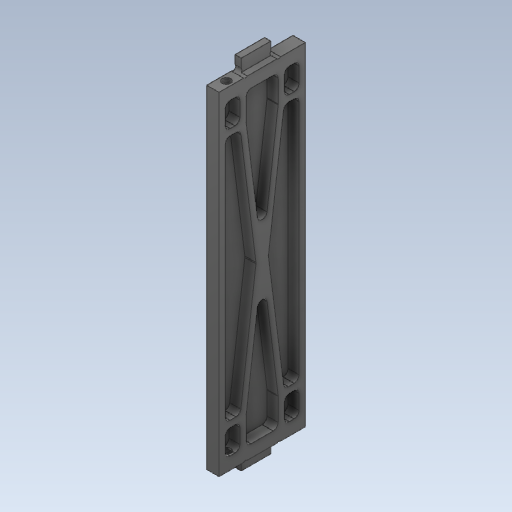
# Autodesk Inventor part: Cockpit_battery_front_frame
Saved by Autodesk Inventor 2020.4 (Build 244396000, 396)
## iProperties
Created: 2022-01-28
Part Number: Cockpit_battery_front_frame
Material: アセタール樹脂、黒
Document SubType Name: Modeling
Designer: Masato Kubotera
Density: 1.425 g/cm^3
Appearance: 滑らか - 黒
Description: POM T5
Author: Masato Kubotera
Autodesk Inventor part; units mm, degrees
ref_plane "XZ Plane" through (0, 0, 0) normal (0, 1, 0) x (-1, 0, 0)
ref_plane "XY Plane" through (0, 0, 0) normal (0, 0, 1) x (1, 0, 0)
derived "Cockpit_side_frame.ipt"
sketch "スケッチ2" plane through (0, 0, 0) normal (0, 1, 0) x (-1, 0, 0)
  line L0 (-28.5, -22.5) -> (88.5, -22.5) construction
  line L1 (88.5, -22.5) -> (88.5, -138.5)
  line L2 (88.5, -96) -> (-28.5, -96) construction
  line L3 (-28.5, -96) -> (-28.5, -22.5) construction
  line L4 (-28.5, -22.5) -> (88.5, -96) construction
  line L5 (88.5, -22.5) -> (-28.5, -96) construction
  line L6 (38.5, -101) -> (38.5, -133.5)
  line L7 (43.5, -138.5) -> (88.5, -138.5)
  arc A0 (64.6349, -63.15) -> (63.15, -64.6349) centre (63.8925, -63.8925) ccw
  arc A1 (73.15, -65.2849) -> (71.6651, -63.8) centre (72.4075, -64.5425) ccw
  line L8 (65.3349, -63.8) -> (71.6651, -63.8)
  line L9 (64.6349, -63.15) -> (72.3651, -63.15)
  line L10 (63.9, -63.85) -> (73.1, -63.85) construction
  arc A2 (65.3349, -63.8) -> (63.85, -65.2849) centre (64.5925, -64.5425) ccw
  line L11 (63.2, -63.2) -> (73.8, -63.2) construction
  line L12 (73.15, -65.2849) -> (73.15, -76.2151)
  line L13 (73.8, -70.75) -> (63.2, -70.75) construction
  line L14 (73.85, -64.6349) -> (73.85, -76.8651)
  line L15 (73.1, -63.85) -> (73.1, -77.65) construction
  line L16 (63.85, -65.2849) -> (63.85, -76.2151)
  line L17 (73.8, -63.2) -> (73.8, -78.3) construction
  line L18 (63.15, -64.6349) -> (63.15, -76.8651)
  line L19 (68.5, -63.2) -> (68.5, -78.3) construction
  line L20 (63.9, -77.65) -> (63.9, -63.85) construction
  line L21 (73.1, -63.85) -> (63.9, -77.65) construction
  line L22 (73.8, -63.2) -> (63.2, -78.3) construction
  line L23 (63.2, -63.2) -> (73.8, -78.3) construction
  line L24 (63.2, -78.3) -> (63.2, -63.2) construction
  line L25 (63.9, -63.85) -> (73.1, -77.65) construction
  arc A3 (73.85, -64.6349) -> (72.3651, -63.15) centre (73.1075, -63.8925) ccw
  line L26 (73.1, -77.65) -> (63.9, -77.65) construction
  line L27 (73.8, -78.3) -> (63.2, -78.3) construction
  arc A4 (63.85, -76.2151) -> (65.3349, -77.7) centre (64.5925, -76.9575) ccw
  arc A5 (63.15, -76.8651) -> (64.6349, -78.35) centre (63.8925, -77.6075) ccw
  line L28 (65.3349, -77.7) -> (71.6651, -77.7)
  line L29 (64.6349, -78.35) -> (72.3651, -78.35)
  arc A6 (71.6651, -77.7) -> (73.15, -76.2151) centre (72.4075, -76.9575) ccw
  arc A7 (72.3651, -78.35) -> (73.85, -76.8651) centre (73.1075, -77.6075) ccw
  line L30 (-23.5, -22.5) -> (-28.5, -27.5)
  line L31 (-28.5, -59.25) -> (88.5, -59.25) construction
  line L32 (30, -22.5) -> (30, -96) construction
  line L33 (-23.5, -96) -> (-28.5, -91)
  line L34 (-28.5, -27.5) -> (-28.5, -91)
  line L35 (-20.5, -24.5) -> (-25.5, -24.5) construction
  line L36 (-25.5, -24.5) -> (-25.5, -94) construction
  line L37 (-25.5, -94) -> (-20.5, -94) construction
  line L38 (-20.5, -94) -> (-20.5, -24.5) construction
  line L39 (-20.5, -24.5) -> (-25.5, -94) construction
  line L40 (-25.5, -24.5) -> (-20.5, -94) construction
  line L41 (-25.55, -46.7) -> (-20.45, -46.7)
  line L42 (-20.45, -46.7) -> (-20.45, -71.8)
  line L43 (-20.45, -71.8) -> (-25.55, -71.8)
  line L44 (-25.55, -71.8) -> (-25.55, -46.7)
  line L45 (-25.55, -46.7) -> (-20.45, -71.8) construction
  line L46 (-20.45, -46.7) -> (-25.55, -71.8) construction
  line L47 (-25.5, -46.75) -> (-20.5, -46.75) construction
  line L48 (-25.5, -71.75) -> (-20.5, -71.75) construction
  line L49 (-23, -24.5) -> (-23, -94) construction
  circle A8 centre (-23, -35) radius 3
  circle A9 centre (-23, -35) radius 1.6
  arc A10 (-24.0651, -46.7) -> (-25.55, -48.1849) centre (-24.8075, -47.4425) ccw
  arc A11 (-20.45, -48.1849) -> (-21.9349, -46.7) centre (-21.1925, -47.4425) ccw
  arc A12 (-21.9349, -71.8) -> (-20.45, -70.3151) centre (-21.1925, -71.0575) ccw
  arc A13 (-25.55, -70.3151) -> (-24.0651, -71.8) centre (-24.8075, -71.0575) ccw
  circle A14 centre (-23, -83.5) radius 1.6
  circle A15 centre (-23, -83.5) radius 3
  line L50 (33.5, -96) -> (38.5, -101)
  line L51 (-23.5, -96) -> (33.5, -96)
  line L52 (81, -46.5) -> (-20.5, -46.5) construction
  line L53 (-20.5, -46.5) -> (-20.5, -41.5) construction
  line L54 (-20.5, -41.5) -> (81, -41.5) construction
  line L55 (81, -41.5) -> (81, -46.5) construction
  line L56 (81, -46.5) -> (-20.5, -41.5) construction
  line L57 (-20.5, -46.5) -> (81, -41.5) construction
  line L58 (-20.5, -44) -> (81, -44) construction
  line L59 (30.25, -41.5) -> (30.25, -46.5) construction
  line L60 (5.25, -41.5) -> (5.25, -46.5) construction
  line L61 (55.3, -41.45) -> (5.2, -41.45)
  line L62 (5.2, -41.45) -> (5.2, -46.55)
  line L63 (5.2, -46.55) -> (55.3, -46.55)
  line L64 (55.3, -46.55) -> (55.3, -41.45)
  line L65 (55.3, -41.45) -> (5.2, -46.55) construction
  line L66 (5.2, -41.45) -> (55.3, -46.55) construction
  arc A16 (6.6849, -41.45) -> (5.2, -42.9349) centre (5.9425, -42.1925) ccw
  circle A17 centre (-2.25, -44) radius 3
  circle A18 centre (-2.25, -44) radius 1.6
  line L67 (55.25, -41.5) -> (55.25, -46.5) construction
  arc A19 (55.3, -42.9349) -> (53.8151, -41.45) centre (54.5575, -42.1925) ccw
  circle A20 centre (62.75, -44) radius 3
  circle A21 centre (62.75, -44) radius 1.6
  arc A22 (5.2, -45.0651) -> (6.6849, -46.55) centre (5.9425, -45.8075) ccw
  arc A23 (53.8151, -46.55) -> (55.3, -45.0651) centre (54.5575, -45.8075) ccw
  line L68 (-20.5, -89) -> (81, -89) construction
  line L69 (81, -89) -> (81, -94) construction
  line L70 (81, -94) -> (-20.5, -94) construction
  line L71 (-20.5, -94) -> (-20.5, -89) construction
  line L72 (-20.5, -89) -> (81, -94) construction
  line L73 (81, -89) -> (-20.5, -94) construction
  line L74 (-20.5, -91.5) -> (81, -91.5) construction
  line L75 (30.25, -89) -> (30.25, -94) construction
  line L76 (55.3, -91.55) -> (5.2, -91.55)
  line L77 (5.2, -91.55) -> (5.2, -88.95)
  line L78 (5.2, -88.95) -> (55.3, -88.95)
  line L79 (55.3, -88.95) -> (55.3, -91.55)
  line L80 (55.3, -91.55) -> (5.2, -88.95) construction
  line L81 (5.2, -91.55) -> (55.3, -88.95) construction
  line L82 (5.25, -89) -> (5.25, -91.5) construction
  line L83 (55.25, -89) -> (55.25, -91.5) construction
  line L84 (5.25, -90.25) -> (55.25, -90.25) construction
  arc A24 (7.3, -88.95) -> (5.2, -88.95) centre (6.25, -88.95) ccw
  arc A25 (55.3, -88.95) -> (53.2, -88.95) centre (54.25, -88.95) ccw
  arc A26 (53.2, -91.55) -> (55.3, -91.55) centre (54.25, -91.55) ccw
  arc A27 (5.2, -91.55) -> (7.3, -91.55) centre (6.25, -91.55) ccw
  circle A28 centre (-2.5, -91.5) radius 3
  circle A29 centre (-2.5, -91.5) radius 1.6
  circle A30 centre (62.5, -91.5) radius 3 construction
  circle A31 centre (62.5, -91.5) radius 1.6 construction
  line L85 (-23.5, -22.5) -> (63.7651, -22.5)
  line L86 (65.25, -21.0151) -> (65.25, -17.5)
  line L87 (65.25, -17.5) -> (73.25, -17.5)
  line L88 (73.25, -17.5) -> (73.25, -21.0151)
  line L89 (81, -22.5) -> (81, -17.5)
  line L90 (88.5, -22.5) -> (88.5, -20)
  line L91 (81, -17.5) -> (86, -17.5)
  line L92 (86, -17.5) -> (88.5, -20)
  line L93 (69.25, -17.5) -> (69.25, -22.5) construction
  arc A32 (63.7651, -22.5) -> (65.25, -21.0151) centre (64.5075, -21.7575) ccw
  arc A33 (73.25, -21.0151) -> (74.7349, -22.5) centre (73.9925, -21.7575) ccw
  arc A34 (79.5151, -22.5) -> (81, -21.0151) centre (80.2575, -21.7575) ccw
  line L94 (-15.5, -89) -> (-15.5, -69) construction
  line L95 (-15.5, -69) -> (64.5, -69) construction
  line L96 (64.5, -69) -> (64.5, -89) construction
  line L97 (45.5, -84) -> (-16.5, -84)
  line L98 (-18.5, -82) -> (-18.5, -63.3955)
  line L99 (-16.5, -61.3955) -> (45.5, -61.3955)
  line L100 (47.5, -63.3955) -> (47.5, -82)
  line L101 (47.5, -84) -> (-18.5, -61.3955) construction
  line L102 (-18.5, -84) -> (47.5, -61.3955) construction
  arc A35 (-16.5, -61.3955) -> (-18.5, -63.3955) centre (-16.5, -63.3955) ccw
  arc A36 (-18.5, -82) -> (-16.5, -84) centre (-16.5, -82) ccw
  arc A37 (45.5, -84) -> (47.5, -82) centre (45.5, -82) ccw
  arc A38 (47.5, -63.3955) -> (45.5, -61.3955) centre (45.5, -63.3955) ccw
  line L103 (38.5, -133.5) -> (43.5, -138.5)
  line L104 (46, -131) -> (41, -131) construction
  line L105 (41, -131) -> (41, -96) construction
  line L106 (41, -96) -> (46, -96) construction
  line L107 (46, -96) -> (46, -131) construction
  line L108 (46, -131) -> (41, -96) construction
  line L109 (41, -131) -> (46, -96) construction
  line L110 (43.5, -96) -> (43.5, -131) construction
  line L111 (41, -113.5) -> (46, -113.5) construction
  line L112 (43.5, -107.5) -> (46, -107.5) construction
  line L113 (43.45, -107.45) -> (46.05, -107.45)
  line L114 (46.05, -107.45) -> (46.05, -119.55)
  line L115 (46.05, -119.55) -> (43.45, -119.55)
  line L116 (43.45, -119.55) -> (43.45, -107.45)
  line L117 (43.45, -107.45) -> (46.05, -119.55) construction
  line L118 (46.05, -107.45) -> (43.45, -119.55) construction
  arc A39 (46.05, -109.55) -> (46.05, -107.45) centre (46.05, -108.5) ccw
  arc A40 (44.9349, -107.45) -> (43.45, -108.9349) centre (44.1925, -108.1925) ccw
  arc A41 (46.05, -119.55) -> (46.05, -117.45) centre (46.05, -118.5) ccw
  line L119 (43.5, -119.5) -> (46, -119.5) construction
  arc A42 (43.45, -118.0651) -> (44.9349, -119.55) centre (44.1925, -118.8075) ccw
  line L120 (44.75, -107.5) -> (44.75, -119.5) construction
  circle A43 centre (43.5, -125.5) radius 3 construction
  circle A44 centre (43.5, -125.5) radius 1.6 construction
  circle A45 centre (43.5, -101.5) radius 3
  circle A46 centre (43.5, -101.5) radius 1.6
  circle A47 centre (-13.5, -55) radius 2
  line L121 (41, -131) -> (79.8645, -131) construction
  line L122 (79.8645, -131) -> (79.8645, -136) construction
  line L123 (79.8645, -136) -> (41, -136) construction
  line L124 (41, -136) -> (41, -131) construction
  line L125 (41, -131) -> (79.8645, -136) construction
  line L126 (79.8645, -131) -> (41, -136) construction
  line L127 (41, -133.5) -> (79.8645, -133.5) construction
  line L128 (60.4322, -131) -> (60.4322, -136) construction
  line L129 (60.4322, -133.5) -> (60.4322, -131) construction
  line L130 (52.8822, -130.95) -> (67.9822, -130.95)
  line L131 (67.9822, -130.95) -> (67.9822, -133.55)
  line L132 (67.9822, -133.55) -> (52.8822, -133.55)
  line L133 (52.8822, -133.55) -> (52.8822, -130.95)
  line L134 (52.8822, -130.95) -> (67.9822, -133.55) construction
  line L135 (67.9822, -130.95) -> (52.8822, -133.55) construction
  line L136 (52.9322, -131) -> (52.9322, -133.5) construction
  arc A48 (54.9822, -130.95) -> (52.8822, -130.95) centre (53.9322, -130.95) ccw
  arc A49 (52.8822, -132.0651) -> (54.3672, -133.55) centre (53.6247, -132.8075) ccw
  arc A50 (67.9822, -130.95) -> (65.8822, -130.95) centre (66.9322, -130.95) ccw
  arc A51 (66.4973, -133.55) -> (67.9822, -132.0651) centre (67.2398, -132.8075) ccw
  line L137 (67.9322, -131) -> (67.9322, -133.5) construction
  line L138 (52.9322, -132.25) -> (67.9322, -132.25) construction
  circle A52 centre (74.4322, -133.5) radius 1.6 construction
  circle A53 centre (74.4322, -133.5) radius 3 construction
  circle A54 centre (46.4322, -133.5) radius 3
  circle A55 centre (46.4322, -133.5) radius 1.6
  line L139 (50.5, -96.5) -> (79, -96.5)
  line L140 (81, -98.5) -> (81, -126.5)
  line L141 (79, -128.5) -> (50.5, -128.5)
  line L142 (48.5, -126.5) -> (48.5, -98.5)
  line L143 (48.5, -96.5) -> (81, -128.5) construction
  line L144 (81, -96.5) -> (48.5, -128.5) construction
  arc A56 (50.5, -96.5) -> (48.5, -98.5) centre (50.5, -98.5) ccw
  arc A57 (48.5, -126.5) -> (50.5, -128.5) centre (50.5, -126.5) ccw
  arc A58 (79, -128.5) -> (81, -126.5) centre (79, -126.5) ccw
  arc A59 (81, -98.5) -> (79, -96.5) centre (79, -98.5) ccw
  line L145 (81, -91.6746) -> (86, -91.6746) construction
  line L146 (86, -91.6746) -> (86, -136) construction
  line L147 (86, -136) -> (81, -136) construction
  line L148 (81, -136) -> (81, -91.6746) construction
  line L149 (81, -91.6746) -> (86, -136) construction
  line L150 (86, -91.6746) -> (81, -136) construction
  line L151 (83.5, -91.6746) -> (83.5, -136) construction
  circle A60 centre (83.5, -94.1746) radius 1.475
  circle A61 centre (83.5, -99.1746) radius 1.475
  circle A62 centre (83.5, -104.1746) radius 1.475
  circle A63 centre (83.5, -133.5) radius 1.6
  arc A64 (86, -91.6746) -> (81, -91.6746) centre (83.5, -133.5) ccw construction
  arc A65 (86.0112, -91.5751) -> (80.9888, -91.5751) centre (83.5, -133.5) ccw construction
  line L152 (88.5, -133.5) -> (83.5, -138.5)
  arc A66 (81, -131) -> (86, -136) centre (83.5, -133.5) ccw construction
  line L153 (86, -91.5) -> (81, -91.5) construction
  circle A67 centre (83.5, -133.5) radius 3
  line L154 (77.125, -22.5) -> (77.125, -27.147) construction
  line L155 (61.375, -22.5) -> (61.375, -27.147) construction
  line L156 (65.25, -22.5) -> (73.25, -22.5)
  line L157 (-18.5, -29.5) -> (-18.5, -34.7517)
  line L158 (-16.5, -36.7517) -> (45.5, -36.7517)
  line L159 (47.5, -34.7517) -> (47.5, -29.5)
  line L160 (45.5, -27.5) -> (-16.5, -27.5)
  arc A68 (-16.5, -27.5) -> (-18.5, -29.5) centre (-16.5, -29.5) ccw
  arc A69 (-18.5, -34.7517) -> (-16.5, -36.7517) centre (-16.5, -34.7517) ccw
  arc A70 (45.5, -36.7517) -> (47.5, -34.7517) centre (45.5, -34.7517) ccw
  arc A71 (47.5, -29.5) -> (45.5, -27.5) centre (45.5, -29.5) ccw
  line L161 (81, -66.9105) -> (86, -66.9105) construction
  line L162 (86, -66.9105) -> (86, -46.9105) construction
  line L163 (86, -46.9105) -> (81, -46.9105) construction
  line L164 (81, -46.9105) -> (81, -66.9105) construction
  line L165 (81, -66.9105) -> (86, -46.9105) construction
  line L166 (86, -66.9105) -> (81, -46.9105) construction
  line L167 (81, -22.5) -> (81, -28.5) construction
  line L168 (81, -28.5) -> (57.5, -28.5) construction
  line L169 (57.5, -28.5) -> (57.5, -22.5) construction
  line L170 (74.7349, -22.5) -> (79.5151, -22.5) construction
  line L171 (74.7349, -22.5) -> (79.5151, -22.5)
  point P0 (0, 0)
  point P1 (30, -59.25)
  point P2 (-25.7227, -96)
  point P3 (63.85, -63.8)
  point P4 (63.15, -63.15)
  point P5 (68.5, -70.75)
  point P6 (-23, -59.25)
  point P7 (30.25, -44)
  point P8 (30.25, -91.5)
  point P9 (30.25, -90.25)
  point P10 (30.25, -90.25)
  point P11 (52.5, -22)
  point P12 (14.5, -72.6978)
  point P13 (-18.5, -61)
  point P14 (47.5, -61)
  point P15 (43.5, -113.5)
  point P16 (44.75, -113.5)
  point P17 (60.4322, -132.25)
  point P18 (64.75, -112.5)
  point P19 (83.5, -113.8373)
  point P20 (-18.5, -36.7517)
  point P21 (47.5, -27.5)
  point P22 (-18.5, -27.5)
  point P23 (73.7349, -22.5)
  point P24 (72.25, -21.0151)
  point P25 (64.4973, -133.55)
  point P26 (63.8822, -130.95)
  point P27 (65.9822, -132.0651)
  point P28 (41.45, -118.0651)
  point P29 (44.05, -117.45)
  point P30 (42.9349, -119.55)
  point P31 (-26.05, -70.3151)
  point P32 (-22.4349, -46.7)
  point P33 (-20.95, -48.1849)
  point P34 (-20.95, -70.3151)
  point P35 (-22.4349, -71.8)
  point P36 (-24.5651, -71.8)
  point P37 (54.05, -59.5651)
  point P38 (52.5651, -61.05)
  point P39 (5.4349, -61.05)
  point P40 (3.95, -59.5651)
  point P41 (52.5651, -55.95)
  point P42 (54.05, -57.4349)
  point P43 (51.95, -88.45)
  point P44 (51.95, -91.05)
  point P45 (6.05, -91.05)
  point P46 (80.4349, -79.8)
  point P47 (78.95, -78.3151)
  point P48 (72.25, -22.5)
  point P49 (83.5, -56.9105)
  point P50 (69.25, -28.5)
  dimension "d1" = 46
  dimension "d2" = 5
  dimension "d3" = 2.5
  measures "d1" horizontal distance of L106.end point (0, 0)
  measures "d2" distance of L106.end L105.end
  measures "d3" distance of L112.start L112.end
ref_plane "作業平面1" through (-46, 0, 0) normal (1, 0, 0) x (0, 1, 0)
sketch "スケッチ3" plane through (-46, 0, 0) normal (1, 0, 0) x (0, 1, 0)
  line L0 (-135, -131) -> (0, -131)
  line L1 (0, -131) -> (0, -96)
  line L2 (0, -96) -> (-135, -96)
  line L3 (-135, -96) -> (-135, -131)
  line L4 (-135, -131) -> (0, -96) construction
  line L5 (0, -131) -> (-135, -96) construction
  line L6 (0, -107.5) -> (5, -107.5)
  line L7 (5, -107.5) -> (5, -119.5)
  line L8 (5, -119.5) -> (0, -119.5)
  line L9 (0, -113.5) -> (-135, -113.5) construction
  line L10 (-67.5, -96) -> (-67.5, -131)
  arc A0 (0, -106.0151) -> (1.4849, -107.5) centre (0.7425, -106.7575) ccw
  line L11 (-7, -98.5) -> (-13, -98.5)
  line L12 (-15, -100.5) -> (-15, -102.5)
  line L13 (-13, -104.5) -> (-7, -104.5)
  line L14 (-5, -102.5) -> (-5, -100.5)
  line L15 (-5, -98.5) -> (-15, -104.5) construction
  line L16 (-15, -98.5) -> (-5, -104.5) construction
  line L17 (-17.5, -100.5) -> (-17.5, -102.8772)
  line L18 (-16.1233, -107) -> (-7, -107)
  line L19 (-5, -109) -> (-5, -118)
  line L20 (-16.3757, -107.016) -> (-51.7468, -111.516)
  line L21 (-67.2476, -110.9679) -> (-19.2476, -104.8612)
  line L22 (-19.5, -98.5) -> (-67.5, -98.5)
  line L23 (-5, -101.5) -> (0, -101.5) construction
  line L24 (-7, -128.5) -> (-13, -128.5)
  line L25 (-15, -126.5) -> (-15, -124.5)
  line L26 (-13, -122.5) -> (-7, -122.5)
  line L27 (-5, -124.5) -> (-5, -126.5)
  line L28 (-17.5, -126.5) -> (-17.5, -124.1228)
  line L29 (-16.1233, -120) -> (-7, -120)
  line L30 (-16.3757, -119.984) -> (-51.7468, -115.484)
  line L31 (-67.2476, -116.0321) -> (-19.2476, -122.1388)
  line L32 (-19.5, -128.5) -> (-67.5, -128.5)
  line L33 (-128, -98.5) -> (-122, -98.5)
  line L34 (-120, -100.5) -> (-120, -102.5)
  line L35 (-122, -104.5) -> (-128, -104.5)
  line L36 (-130, -102.5) -> (-130, -100.5)
  line L37 (-117.5, -100.5) -> (-117.5, -102.8772)
  line L38 (-118.8767, -107) -> (-128, -107)
  line L39 (-130, -109) -> (-130, -118)
  line L40 (-118.6243, -107.016) -> (-83.2532, -111.516)
  line L41 (-67.7524, -110.9679) -> (-115.7524, -104.8612)
  line L42 (-115.5, -98.5) -> (-67.5, -98.5)
  line L43 (-128, -128.5) -> (-122, -128.5)
  line L44 (-130, -124.5) -> (-130, -126.5)
  line L45 (-122, -122.5) -> (-128, -122.5)
  line L46 (-120, -126.5) -> (-120, -124.5)
  line L47 (-117.5, -126.5) -> (-117.5, -124.1228)
  line L48 (-115.5, -128.5) -> (-67.5, -128.5)
  line L49 (-67.7524, -116.0321) -> (-115.7524, -122.1388)
  line L50 (-118.6243, -119.984) -> (-83.2532, -115.484)
  line L51 (-118.8767, -120) -> (-128, -120)
  arc A1 (-5, -100.5) -> (-7, -98.5) centre (-7, -100.5) ccw
  arc A2 (-13, -98.5) -> (-15, -100.5) centre (-13, -100.5) ccw
  arc A3 (-15, -102.5) -> (-13, -104.5) centre (-13, -102.5) ccw
  arc A4 (-7, -104.5) -> (-5, -102.5) centre (-7, -102.5) ccw
  arc A5 (-19.2476, -104.8612) -> (-17.5, -102.8772) centre (-19.5, -102.8772) ccw
  arc A6 (-17.5, -100.5) -> (-19.5, -98.5) centre (-19.5, -100.5) ccw
  arc A7 (-115.5, -98.5) -> (-117.5, -100.5) centre (-115.5, -100.5) ccw
  arc A8 (-117.5, -102.8772) -> (-115.7524, -104.8612) centre (-115.5, -102.8772) ccw
  arc A9 (-67.7524, -110.9679) -> (-67.2476, -110.9679) centre (-67.5, -108.9839) ccw
  arc A10 (-51.7468, -111.516) -> (-51.7468, -115.484) centre (-51.4944, -113.5) ccw
  arc A11 (-16.1233, -107) -> (-16.3757, -107.016) centre (-16.1233, -109) ccw
  arc A12 (-5, -109) -> (-7, -107) centre (-7, -109) ccw
  arc A13 (-7, -120) -> (-5, -118) centre (-7, -118) ccw
  arc A14 (-16.3757, -119.984) -> (-16.1233, -120) centre (-16.1233, -118) ccw
  arc A15 (-13, -122.5) -> (-15, -124.5) centre (-13, -124.5) ccw
  arc A16 (-15, -126.5) -> (-13, -128.5) centre (-13, -126.5) ccw
  arc A17 (-7, -128.5) -> (-5, -126.5) centre (-7, -126.5) ccw
  arc A18 (-5, -124.5) -> (-7, -122.5) centre (-7, -124.5) ccw
  arc A19 (-19.5, -128.5) -> (-17.5, -126.5) centre (-19.5, -126.5) ccw
  arc A20 (-17.5, -124.1228) -> (-19.2476, -122.1388) centre (-19.5, -124.1228) ccw
  arc A21 (-67.2476, -116.0321) -> (-67.7524, -116.0321) centre (-67.5, -118.0161) ccw
  arc A22 (-122, -128.5) -> (-120, -126.5) centre (-122, -126.5) ccw
  arc A23 (-120, -124.5) -> (-122, -122.5) centre (-122, -124.5) ccw
  arc A24 (-128, -122.5) -> (-130, -124.5) centre (-128, -124.5) ccw
  arc A25 (-130, -126.5) -> (-128, -128.5) centre (-128, -126.5) ccw
  arc A26 (-117.5, -126.5) -> (-115.5, -128.5) centre (-115.5, -126.5) ccw
  arc A27 (-115.7524, -122.1388) -> (-117.5, -124.1228) centre (-115.5, -124.1228) ccw
  arc A28 (-130, -118) -> (-128, -120) centre (-128, -118) ccw
  arc A29 (-128, -107) -> (-130, -109) centre (-128, -109) ccw
  arc A30 (-118.6243, -107.016) -> (-118.8767, -107) centre (-118.8767, -109) ccw
  arc A31 (-83.2532, -115.484) -> (-83.2532, -111.516) centre (-83.5056, -113.5) ccw
  arc A32 (-130, -102.5) -> (-128, -104.5) centre (-128, -102.5) ccw
  arc A33 (-128, -98.5) -> (-130, -100.5) centre (-128, -100.5) ccw
  arc A34 (-120, -100.5) -> (-122, -98.5) centre (-122, -100.5) ccw
  arc A35 (-122, -104.5) -> (-120, -102.5) centre (-122, -102.5) ccw
  arc A36 (-118.8767, -120) -> (-118.6243, -119.984) centre (-118.8767, -118) ccw
  arc A37 (1.4849, -119.5) -> (0, -120.9849) centre (0.7425, -120.2425) ccw
  point P0 (0, 0)
  point P1 (-67.5, -113.5)
  point P2 (0, -107.5)
  point P3 (0, -107.5)
  point P4 (0, -107.5)
  point P5 (0, -119.5)
  point P6 (0, -119.5)
  point P7 (0, -119.5)
  point P8 (-10, -101.5)
  point P9 (-17.5, -98.5)
  point P10 (-16.25, -107)
  point P11 (-5, -107)
  point P12 (-67.3416, -113.5)
  point P13 (-67.5, -111)
  point P14 (-17.5, -104.6389)
  point P15 (-5, -128.5)
  point P16 (-15, -122.5)
  point P17 (-15, -128.5)
  point P18 (-5, -122.5)
  point P19 (-17.5, -128.5)
  point P20 (-16.25, -120)
  point P21 (-5, -120)
  point P22 (-67.5, -116)
  point P23 (-17.5, -122.3611)
  point P24 (-130, -98.5)
  point P25 (-120, -104.5)
  point P26 (-120, -98.5)
  point P27 (-130, -104.5)
  point P28 (-117.5, -98.5)
  point P29 (-118.75, -107)
  point P30 (-130, -107)
  point P31 (-67.6584, -113.5)
  point P32 (-117.5, -104.6389)
  point P33 (-130, -128.5)
  point P34 (-120, -128.5)
  point P35 (-130, -122.5)
  point P36 (-120, -122.5)
  point P37 (-117.5, -128.5)
  point P38 (-117.5, -122.3611)
  point P39 (-118.75, -120)
  point P40 (-130, -120)
  point P41 (-67.5, -110.9839)
  point P42 (-67.5, -116.0161)
  point P43 (0, -120.9849)
  point P44 (1.4849, -119.5)
  dimension "d5" = 1.05
  dimension "d6" = 5
  dimension "d7" = 135
  dimension "d8" = 2.5
  dimension "d9" = 2.5
  dimension "d10" = 5
  dimension "d11" = 2.5
  dimension "d14" = 5
  dimension "d15" = 2
  dimension "d16" = 10
  dimension "d17" = 2.5
  dimension "d18" = 11.25
  constraints: 104 end point, 79 point on line, 77 point on circle, 72 tangent, 38 centre point, 35 equal radius, 30 symmetric about line, 9 midpoint, 8 perpendicular, 5 parallel, 4 coincident, 3 horizontal, 2 collinear, 1 vertical, 1 other
  measures "d5" radius of A0
  measures "d6" distance of L6.start L6.end
  measures "d7" distance of L1.end L2.end
  measures "d8" vertical distance of L15.start L1.end
  measures "d9" distance of point (-5, -107) L16.end
  measures "d10" horizontal distance of L15.start L1.end
  measures "d11" distance of point (-17.5, -98.5) L16.start
  measures "d14" distance of point (-67.5, -116) point (-67.5, -111)
  measures "d15" radius of A1
  measures "d16" distance of L15.start L16.start
  measures "d17" distance between parallel lines of L21 L20
  measures "d18" distance of point (-5, -107) point (-16.25, -107)
extrude "押し出し1" add sketch "スケッチ3" along normal blind 5 contours L10 L32 A19 L28 A20 L31 A21 A9 L21 A5 L17 A6 L22 L2 L1 A0 A37 L0
extrude "押し出し2" add sketch "スケッチ3" along normal blind 2.5 contours L1 A0 L6 L7 L8 A37
extrude "押し出し3" add sketch "スケッチ3" along normal blind 0.5 contours L10 A21 L31 A20 L28 A19 L32 | L22 A6 L17 A5 L21 A9 L10 | A1 L14 A4 L13 A3 L12 A2 L11 | L18 A12 L19 A13 L29 A14 L30 A10 L20 A11 | L24 A16 L25 A15 L26 A18 L27 A17
hole "穴1" at (-43.5, 0, -101.5) direction (0, -1, 0) diameter 3.4587 depth 5 thread size "M4x0.5" class "6H" standard "ISO Metric profile"
mirror "ミラー1" about plane through (-46, -67.5, -128.5) normal (0, -1, 0)
equation "\"d9\" = d8"
equation "\"d11\" = d8"
equation "\"d18\" = d16 + 0.5 * d11"
equation "\"d19\" = d2"
equation "\"d21\" = d3"
equation "\"d4\" = -d1"
